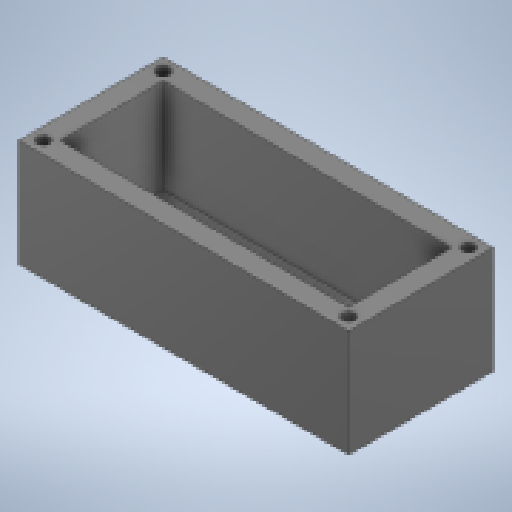
# Autodesk Inventor part: camera_case_2
Saved by Autodesk Inventor 2026.2 (Build 302298010, 298A)
## iProperties
Created: 2026-05-11
Part Number: camera_case_2
Material: ABS Plastic
Document SubType Name: Modeling
Designer: chris
Density: 1.06 g/cm^3
Appearance: Smooth - White
Author: chris
Autodesk Inventor part; units mm, degrees
ref_plane "YZ Plane" through (0, 0, 0) normal (1, 0, 0) x (0, 1, 0)
ref_plane "XZ Plane" through (0, 0, 0) normal (0, 1, 0) x (-1, 0, 0)
ref_plane "XY Plane" through (0, 0, 0) normal (0, 0, 1) x (1, 0, 0)
sketch "Sketch1" plane through (0, 0, 0) normal (0, 1, 0) x (-1, 0, 0)
  line L0 (40, 17.5) -> (-40, 17.5)
  line L1 (-40, 17.5) -> (-40, -17.5)
  line L2 (-40, -17.5) -> (40, -17.5)
  line L3 (40, -17.5) -> (40, 17.5)
  line L4 (40, 17.5) -> (-40, -17.5) construction
  line L5 (-40, 17.5) -> (40, -17.5) construction
  point P0 (0, 0)
  dimension "d0" = 80
  dimension "d1" = 35
  constraints: 12 end point, 2 midpoint, 2 parallel, 1 horizontal, 1 perpendicular
  measures "d0" distance of L2.end L1.end
  measures "d1" distance of L1.end L0.end
extrude "Extrusion1" add sketch "Sketch1" along normal blind 3
sketch "Sketch2" plane through (0, 3, 0) normal (0, 1, 0) x (1, 0, 0)
  line L0 (35, -12.5) -> (-35, -12.5)
  line L1 (-35, -12.5) -> (-35, 12.5)
  line L2 (-35, 12.5) -> (35, 12.5)
  line L3 (35, 12.5) -> (35, -12.5)
  line L4 (35, -12.5) -> (-35, 12.5) construction
  line L5 (-35, -12.5) -> (35, 12.5) construction
  line L6 (40, 17.5) -> (-40, 17.5) projected
  line L7 (40, -17.5) -> (40, 17.5) projected
  line L8 (40, -17.5) -> (40, 17.5) projected
  line L9 (40, 17.5) -> (-40, 17.5) projected
  line L10 (-40, 17.5) -> (-40, -17.5) projected
  line L11 (-40, -17.5) -> (40, -17.5) projected
  point P0 (0, 0)
  dimension "d4" = 70
  dimension "d5" = 25
  constraints: 12 end point, 2 midpoint, 2 parallel, 1 horizontal, 1 perpendicular
  measures "d4" distance of L1.end L2.end
  measures "d5" distance of L0.end L1.end
extrude "Extrusion2" add sketch "Sketch2" along normal blind 23
sketch "Sketch3" plane through (0, 26, 0) normal (0, 1, 0) x (1, 0, 0)
  circle A0 centre (-37, -14.5) radius 1.5
  line L0 (-40, 17.5) -> (-40, -17.5) projected
  line L1 (-40, -17.5) -> (40, -17.5) projected
  circle A1 centre (-37, 14.5) radius 1.5
  circle A2 centre (37, 14.5) radius 1.5
  circle A3 centre (37, -14.5) radius 1.5
  line L2 (40, 17.5) -> (-40, 17.5) projected
  line L3 (40, -17.5) -> (40, 17.5) projected
  point P0 (0, 0)
  dimension "d11" = 3
  dimension "d12" = 3
  dimension "d13" = 3
  dimension "d14" = 3
  dimension "d15" = 3
  dimension "d16" = 3
  dimension "d17" = 3
  dimension "d18" = 3
  dimension "d19" = 3
  dimension "d20" = 3
  dimension "d21" = 3
  dimension "d22" = 3
  constraints: 4 centre point
  measures "d11" diameter of A0
  measures "d12" distance from line of L0 A0.centre
  measures "d13" distance from line of L1 A0.centre
  measures "d14" diameter of A1
  measures "d15" diameter of A2
  measures "d16" diameter of A3
  measures "d17" distance from line of L2 A1.centre
  measures "d18" distance from line of A1.centre L0
  measures "d19" distance from line of L3 A2.centre
  measures "d20" distance from line of L2 A2.centre
  measures "d21" distance from line of L1 A3.centre
  measures "d22" distance from line of L3 A3.centre
extrude "Extrusion3" cut sketch "Sketch3" against normal through all contours A0 | A1 | A2 | A3
sketch "Sketch4" plane through (0, 0, 0) normal (0, -1, 0) x (1, 0, 0)
  circle A0 centre (0, 0) radius 10
  dimension "d25" = 20
  constraints: 1 centre point, 1 coincident
  measures "d25" diameter of A0
extrude "Extrusion4" cut sketch "Sketch4" against normal blind 10
body "Solid1"
